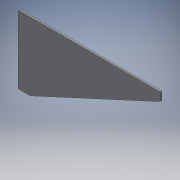
# Autodesk Inventor part: Projector mount side
Saved by Autodesk Inventor 2019 (Build 230136000, 136)
## iProperties
Created: 2020-03-21
Part Number: Projector mount side
Material: Generic
Document SubType Name: Modeling
Designer: Vijay
Density: 1 g/cm^3
Appearance: Default
Author: Vijay
Autodesk Inventor part; units mm, degrees
ref_plane "YZ Plane" through (0, 0, 0) normal (1, 0, 0) x (0, 1, 0)
ref_plane "XZ Plane" through (0, 0, 0) normal (0, 1, 0) x (-1, 0, 0)
ref_plane "XY Plane" through (0, 0, 0) normal (0, 0, 1) x (1, 0, 0)
sketch "Sketch1" plane through (0, 0, 0) normal (0, 0, 1) x (1, 0, 0)
  line L0 (11.9, 0) -> (6, 0) construction
  line L1 (6, 4) -> (11.9, 4) construction
  line L2 (-150.8, -316.8297) -> (-150.8003, 183.1703) construction
  line L3 (210, 14) -> (-150.8001, 14)
  line L4 (-150.8001, 14) -> (-150.8001, -160)
  line L5 (-150.8001, -160) -> (-120.8001, -160)
  line L6 (210, -7.5086) -> (210, 14)
  line L7 (-120.8, -316.8296) -> (-120.8003, 183.1704) construction
  line L8 (-120.8001, -160) -> (210, -7.5086)
  line L9 (425, -160) -> (0, -160) projected
  line L10 (6, 4) -> (6, 0) projected
  line L11 (11.9, 0) -> (11.9, 4) projected
  dimension "d0" = 10
  constraints: 10 end point, 2 parallel, 2 point on line, 1 collinear, 1 horizontal, 1 perpendicular
  measures "d0" distance between parallel lines of L3 L1
extrude "Extrusion1" add sketch "Sketch1" along normal blind 4
fillet "Fillet1" radius 2 5 edges at (210, 14, 2) (210, -7.5086, 2) (-150.8001, 14, 2) (-150.8001, -160, 2) (-120.8001, -160, 2)
sketch "Sketch2" plane through (0, 0, 4) normal (0, 0, 1) x (1, 0, 0)
  point P0 (0, 0)
sketch "Sketch3" plane through (0, 0, 4) normal (0, 0, 1) x (1, 0, 0)
  line L0 (200, 0) -> (200, 4) projected
  line L1 (200, 4) -> (199.5, 4) projected
  line L2 (194.5, 4) -> (199.5, 4) projected
  line L3 (194.5, 4) -> (194, 4) projected
  line L4 (194, 0) -> (194, 4)
  line L5 (194, 0) -> (194.5, 0) projected
  line L6 (199.5, 0) -> (194.5, 0) projected
  line L7 (199.5, 0) -> (200, 0) projected
  line L8 (200.2, 4.2) -> (200.2, -0.2)
  line L9 (200.2, -0.2) -> (199.5, -0.2)
  line L10 (199.5, -0.2) -> (194.5, -0.2)
  line L11 (194.5, -0.2) -> (193.8, -0.2)
  line L12 (193.8, -0.2) -> (193.8, 4.2)
  line L13 (193.8, 4.2) -> (194.5, 4.2)
  line L14 (194.5, 4.2) -> (199.5, 4.2)
  line L15 (199.5, 4.2) -> (200.2, 4.2)
  line L16 (178.3, 0) -> (173.3, 0) projected
  line L17 (178.3, 0) -> (178.8, 0) projected
  line L18 (178.8, 0) -> (178.8, 4) projected
  arc A0 (-121.2388, -160) -> (-120.4016, -159.8163) centre (-121.2388, -158) ccw projected
  line L19 (-120.4016, -159.8163) -> (208.8373, -8.0446) projected
  arc A1 (208.8373, -8.0446) -> (210, -6.2283) centre (208, -6.2283) ccw projected
  line L20 (210, -6.2283) -> (210, 12) projected
  arc A2 (210, 12) -> (208, 14) centre (208, 12) ccw projected
  line L21 (208, 14) -> (-148.8001, 14) projected
  arc A3 (-148.8001, 14) -> (-150.8001, 12) centre (-148.8001, 12) ccw projected
  line L22 (-150.8001, 12) -> (-150.8001, -158) projected
  arc A4 (-150.8001, -158) -> (-148.8001, -160) centre (-148.8001, -158) ccw projected
  line L23 (-148.8001, -160) -> (-121.2388, -160) projected
  line L24 (178.8, 4) -> (178.3, 4) projected
  line L25 (173.3, 4) -> (178.3, 4) projected
  line L26 (173.3, 4) -> (172.8, 4) projected
  line L27 (172.8, 0) -> (172.8, 4) projected
  line L28 (172.8, 0) -> (173.3, 0) projected
  line L29 (21.7, 4) -> (26.7, 4) projected
  line L30 (27.2, 4) -> (26.7, 4) projected
  line L31 (27.2, 0) -> (27.2, 4)
  line L32 (26.7, 0) -> (27.2, 0) projected
  line L33 (26.7, 0) -> (21.7, 0) projected
  line L34 (21.2, 0) -> (21.7, 0) projected
  line L35 (21.2, 0) -> (21.2, 4)
  line L36 (21.7, 4) -> (21.2, 4) projected
  line L37 (6, 0) -> (6, 4)
  line L38 (0, 0) -> (0, 4) projected
  line L39 (5.5, 0) -> (0.5, 0) projected
  line L40 (0.5, 4) -> (5.5, 4) projected
  line L41 (6, 4) -> (5.5, 4) projected
  line L42 (5.5, 0) -> (6, 0) projected
  line L43 (0, 0) -> (0.5, 0) projected
  line L44 (0.5, 4) -> (0, 4) projected
  line L45 (11.9, 4) -> (15.3, 4) projected
  line L46 (11.9, 4) -> (11.9, 0) projected
  line L47 (15.3, 0) -> (11.9, 0) projected
  line L48 (15.3, 4) -> (15.3, 0) projected
  line L49 (184.7, 4) -> (188.1, 4) projected
  line L50 (184.7, 4) -> (184.7, 0) projected
  line L51 (188.1, 0) -> (184.7, 0) projected
  line L52 (188.1, 4) -> (188.1, 0) projected
  line L53 (179, 4.2) -> (179, -0.2)
  line L54 (179, -0.2) -> (178.3, -0.2)
  line L55 (178.3, -0.2) -> (173.3, -0.2)
  line L56 (173.3, -0.2) -> (172.6, -0.2)
  line L57 (172.6, -0.2) -> (172.6, 4.2)
  line L58 (172.6, 4.2) -> (173.3, 4.2)
  line L59 (173.3, 4.2) -> (178.3, 4.2)
  line L60 (178.3, 4.2) -> (179, 4.2)
  line L61 (21.7, -0.2) -> (26.7, -0.2)
  line L62 (26.7, -0.2) -> (27.4, -0.2)
  line L63 (27.4, -0.2) -> (27.4, 4.2)
  line L64 (27.4, 4.2) -> (26.7, 4.2)
  line L65 (26.7, 4.2) -> (21.7, 4.2)
  line L66 (21.7, 4.2) -> (21, 4.2)
  line L67 (21, 4.2) -> (21, -0.2)
  line L68 (21, -0.2) -> (21.7, -0.2)
  line L69 (-0.2, 4.2) -> (-0.2, -0.2)
  line L70 (-0.2, -0.2) -> (0.5, -0.2)
  line L71 (0.5, -0.2) -> (5.5, -0.2)
  line L72 (5.5, -0.2) -> (6.2, -0.2)
  line L73 (6.2, -0.2) -> (6.2, 4.2)
  line L74 (6.2, 4.2) -> (5.5, 4.2)
  line L75 (5.5, 4.2) -> (0.5, 4.2)
  line L76 (0.5, 4.2) -> (-0.2, 4.2)
  circle A5 centre (13.6, 2) radius 1.6
  circle A6 centre (186.4, 2) radius 1.6
  point P0 (0, 0)
  dimension "d5" = 0.2
  dimension "d6" = 0.2
  dimension "d7" = 0.2
  dimension "d8" = 0.2
  dimension "d9" = 3.2
  dimension "d10" = 3.2
  constraints: 72 end point, 4 vertical, 2 centre point, 33 other
  measures "d5" distance between parallel lines of L0 L8
  measures "d6" distance between parallel lines of L18 L53
  measures "d7" distance between parallel lines of L33 L61
  measures "d8" distance between parallel lines of L38 L69
  measures "d9" diameter of A5
  measures "d10" diameter of A6
extrude "Extrusion2" cut sketch "Sketch3" against normal blind 4 contours L7 L6 L5 L4 L3 L2 L1 L0 | L8 L9 L10 L11 L12 L13 L14 L15 | L16 L28 L27 L26 L25 L24 L18 L17 | L29 L30 L31 L32 L33 L34 L35 L36 | L42 L39 L43 L38 L44 L40 L41 L37 | L53 L54 L55 L56 L57 L58 L59 L60 | L68 L67 L66 L65 L64 L63 L62 L61 | L76 L75 L74 L73 L72 L71 L70 L69 | A5 | A6
sketch "Sketch4" plane through (0, 0, 4) normal (0, 0, 1) x (1, 0, 0)
  line L0 (-139.9, -316.8296) -> (-139.9003, 183.1704) construction
  line L1 (-131.7, -316.8296) -> (-139.9, -316.8296) construction
  line L2 (-131.7, -316.8296) -> (-131.7003, 183.1704) construction
  line L3 (-139.9003, 183.1704) -> (-131.7003, 183.1704) construction
  line L4 (-131.7002, 4) -> (-139.9001, 4) construction
  line L5 (-139.9001, 4) -> (-139.9001, -150) construction
  line L6 (-139.9001, -150) -> (-131.7002, -150) construction
  line L7 (-131.7002, -150) -> (-131.7002, 4) construction
  line L8 (208, 14) -> (-148.8001, 14) projected
  line L9 (-148.8001, -160) -> (-121.2388, -160) projected
  circle A0 centre (-135.8001, 4) radius 2.5
  circle A1 centre (-135.8001, -150) radius 2.5
  point P0 (0, 0)
  dimension "d13" = 10
  dimension "d14" = 10
  dimension "d15" = 5
  dimension "d16" = 5
  constraints: 8 end point, 2 centre point, 2 midpoint, 2 parallel, 2 point on line, 1 horizontal, 1 perpendicular
  measures "d13" distance between parallel lines of L8 L4
  measures "d14" distance between parallel lines of L6 L9
  measures "d15" diameter of A0
  measures "d16" diameter of A1
extrude "Extrusion3" cut sketch "Sketch4" against normal blind 4
body "Solid1"
